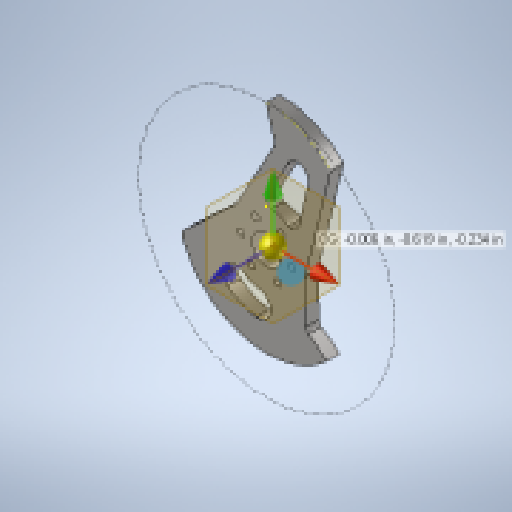
# Autodesk Inventor part: Blade
Saved by Autodesk Inventor 2023.4 (Build 274418000, 418)
## iProperties
Created: 2023-11-12
Part Number: Blade
Material: Steel, Alloy
Document SubType Name: Modeling
Designer: Nathan Cai
Density: 7.73 g/cm^3
Appearance: Semi-Polished
Mass: 170.251 g
Surface Area: 105.152 cm^2
Volume: 22.0248 cm^3
Author: Nathan Cai
Autodesk Inventor part; units mm, degrees
ref_plane "YZ Plane" through (0, 0, 0) normal (1, 0, 0) x (0, 1, 0)
ref_plane "XZ Plane" through (0, 0, 0) normal (0, 1, 0) x (-1, 0, 0)
ref_plane "XY Plane" through (0, 0, 0) normal (0, 0, 1) x (1, 0, 0)
sketch "Sketch1" plane through (0, 0, 0) normal (0, 0, 1) x (1, 0, 0)
  circle A0 centre (0, 0) radius 63.5 construction
  circle A1 centre (0, 0) radius 7.1437
  circle A2 centre (0, 0) radius 12.7 construction
  circle A3 centre (0, 0) radius 19.05
  line L0 (0, 63.5) -> (0, 0) construction
  line L1 (0, 63.5) -> (4.306, 47.4299)
  line L2 (4.306, 47.4299) -> (-16.6992, 9.1674)
  circle A4 centre (0, 0) radius 47.625 construction
  arc A5 (31.8711, 50.0344) -> (0, 63.5) centre (0, 19.05) ccw
  line L3 (31.8711, 50.0344) -> (18.5028, -4.533)
  circle A6 centre (0, 0) radius 44.45 construction
  line L4 (30.03, -32.772) -> (0, 0) construction
  line L5 (30.03, -32.772) -> (19.7345, -24.8719)
  line L6 (19.7345, -24.8719) -> (19.0429, 0.5186)
  circle A7 centre (0, 0) radius 31.75 construction
  arc A8 (-42.3927, -13.3664) -> (30.03, -32.772) centre (0, 0) ccw
  line L7 (-42.3927, -13.3664) -> (-12.9621, 13.9602)
  line L8 (-42.3927, -13.3664) -> (0, 0) construction
  line L9 (-2.2951, 18.9112) -> (10.5685, 42.3434)
  line L10 (14.4751, 12.3844) -> (20.8358, 38.3475)
  arc A9 (20.8358, 38.3475) -> (10.5685, 42.3434) centre (15.4391, 39.6696) ccw
  line L11 (-10.9985, 6.35) -> (0, 0) construction
  line L12 (0, 0) -> (-5.3673, 11.5101) construction
  circle A10 centre (-5.3673, 11.5101) radius 1.7526
  circle A11 centre (-12.6517, 1.1069) radius 1.7526
  circle A12 centre (-7.2844, -10.4032) radius 1.7526
  circle A13 centre (5.3673, -11.5101) radius 1.7526
  circle A14 centre (12.6517, -1.1069) radius 1.7526
  circle A15 centre (7.2844, 10.4032) radius 1.7526
  arc A16 (-15.4432, -20.166) -> (-4.1463, -25.0593) centre (0, 0) ccw construction
  arc A17 (-19.304, -25.2075) -> (-5.1829, -31.3241) centre (0, 0) ccw
  arc A18 (-11.5824, -15.1245) -> (-3.1097, -18.7945) centre (0, 0) ccw
  arc A19 (-11.5824, -15.1245) -> (-19.304, -25.2075) centre (-15.4432, -20.166) ccw
  arc A20 (-5.1829, -31.3241) -> (-3.1097, -18.7945) centre (-4.1463, -25.0593) ccw
  line L13 (-15.4432, -20.166) -> (0, 0) construction
  line L14 (-4.1463, -25.0593) -> (0, 0) construction
  line L15 (0, 0) -> (-10.0957, -23.3074) construction
  point P0 (19.1127, -2.0435)
  point P1 (-15.2178, 11.8657)
  point P2 (-3.1097, -18.7945)
  dimension "d0" = 127
  dimension "d8" = 38.1
  dimension "d14" = 15.875
  dimension "d17" = 63.5
  dimension "d1" = 14.2875
  dimension "d2" = 25.4
  dimension "d9" = 15
  dimension "d11" = 44.45
  dimension "d12" = 15
  dimension "d15" = 88.9
  dimension "d16" = 10
  dimension "d18" = 42.5
  dimension "d19" = 115
  dimension "d28" = 7.9375
  dimension "d29" = 7.9375
  dimension "d30" = 5.5563
  dimension "d31" = 35
  dimension "d32" = 3.5052
  dimension "d35" = 360
  dimension "d40" = 60
  dimension "d41" = 12.7
  dimension "d43" = 28.05
  dimension "d44" = 156.58
  constraints: 32 end point, 21 point on circle, 17 centre point, 9 coincident, 6 tangent, 2 concentric, 2 parallel, 1 vertical, 1 vertical alignment, 35 other
  measures "d1" diameter of A1
  measures "d2" diameter of A2
  measures "d9" angle of L0 L1
  measures "d11" radius of A5
  measures "d12" angle of L2 L3
  measures "d15" diameter of A6
  measures "d16" angle of L4 L5
  measures "d18" angle of L0 L4
  measures "d19" angle of L4 L8
  measures "d28" distance between parallel lines of L3 L10
  measures "d29" distance between parallel lines of L2 L9
  measures "d30" radius of A9
  measures "d31" angle of L11 L12
  measures "d32" diameter of A10
  measures "d40" angle of L0 L11
  measures "d41" diameter of A20
  measures "d43" angle of L13 L14
  measures "d44" angle of L15 L0
extrude "Extrusion1" add sketch "Sketch1" along normal blind 6.35 contours A3 | A3 L6 L3 | A3 L10 A9 L9 L7 L2 L1 A5 L3 L6 | L3 L6 L5 A8 L7 L2 A3 A19 A17 A20 | A3 L2 L7
fillet "Fillet1" radius 3.175 6 edges at (19.1127, -2.0435, 3.175) (19.7345, -24.8719, 3.175) (4.306, 47.4299, 3.175) (-2.2951, 18.9112, 3.175) (14.4751, 12.3844, 3.175) (-15.2178, 11.8657, 3.175)
fillet "Fillet3" radius 3.175 1 edges at (-42.3927, -13.3664, 3.175)
sketch "Sketch2" plane through (0, 0, 6.35) normal (0, 0, 1) x (1, 0, 0)
  arc A0 (31.8711, 50.0344) -> (0, 63.5) centre (0, 19.05) ccw construction
  circle A1 centre (0, 0) radius 63.5 construction
  constraints: 1 coincident, 1 vertical alignment, 2 other
equation "\"d29\" = d28"
body "Solid1"
